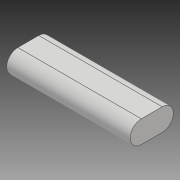
# Autodesk Inventor part: battery
Saved by Autodesk Inventor 2018 (Build 220112000, 112)
## iProperties
Created: 2019-02-20
Part Number: battery
Material: 一般
Document SubType Name: Modeling
Designer: ku_sk
Density: 1 g/cm^3
Appearance: 既定
Author: ku_sk
Autodesk Inventor part; units mm, degrees
ref_plane "YZ Plane" through (0, 0, 0) normal (1, 0, 0) x (0, 1, 0)
ref_plane "XZ Plane" through (0, 0, 0) normal (0, 1, 0) x (-1, 0, 0)
ref_plane "XY Plane" through (0, 0, 0) normal (0, 0, 1) x (1, 0, 0)
sketch "スケッチ1" plane through (0, 0, 0) normal (1, 0, 0) x (0, 1, 0)
  line L0 (11.5, 0) -> (-11.5, 0) construction
  line L1 (11.5, 12.25) -> (-11.5, 12.25)
  line L2 (-11.5, -12.25) -> (11.5, -12.25)
  arc A0 (11.5, -12.25) -> (11.5, 12.25) centre (11.5, 0) ccw
  arc A1 (-11.5, 12.25) -> (-11.5, -12.25) centre (-11.5, 0) ccw
  point P0 (0, 0)
  point P1 (0, 0)
  point P2 (23.75, 0)
  point P3 (-23.75, 0)
  dimension "d0" = 24.5
  dimension "d1" = 47.5
  constraints: 8 end point, 6 point on circle, 4 tangent, 2 centre point, 1 coincident, 1 horizontal, 1 midpoint, 1 parallel
  measures "d0" distance between parallel lines of L2 L1
  measures "d1" distance of point (-23.75, 0) point (23.75, 0)
extrude "押し出し1" add sketch "スケッチ1" along normal mid plane 136
